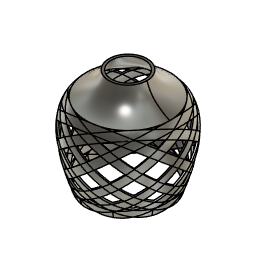
Design a 3D Printed Lampshade_ (Autodesk Fusion 360 design; units mm, degrees)
Autodesk Fusion 360 part; units mm, degrees
sketch "Sketch1" plane through (0, 0, 0) normal (0, 1, 0) x (1, 0, 0)
  line L0 (0, 0) -> (-45, 0)
  line L1 (0, -135) -> (-23.4, -135)
  spline S0 degree 5 poles (-45, 0) (-46.977, -5.2113) (-50.6671, -15.359) (-55.4104, -29.7559) (-60.125, -47.2752) (-63.1831, -66.2213) (-63.2423, -82.0437) (-60.2343, -94.6701) (-54.3436, -104.2914) (-46.1941, -111.555) (-37.1505, -117.879) (-30.513, -123.5506) (-26.5029, -128.8056) (-24.3479, -132.8457) (-23.4, -135) knots 0 0 0 0 0 0 0.1 0.2 0.3 0.4 0.5 0.6 0.7 0.8 0.9 1 1 1 1 1 1
  line L2 (-30, -120) -> (-16.8, -150)
  spline S1 degree 5 poles (-45, 0) (-46.977, -5.2113) (-50.6671, -15.359) (-55.4104, -29.7559) (-60.125, -47.2752) (-63.1831, -66.2213) (-63.2423, -82.0437) (-60.2343, -94.6701) (-54.3436, -104.2914) (-46.1941, -111.555) (-37.1505, -117.879) (-30.513, -123.5506) (-26.5029, -128.8056) (-24.3479, -132.8457) (-23.4, -135) knots 0 0 0 0 0 0 0.1 0.2 0.3 0.4 0.5 0.6 0.7 0.8 0.9 1 1 1 1 1 1
  line L3 (-30, -120) -> (-16.8, -150)
  spline S2 degree 5 poles (-43, 0) (-44.977, -5.2113) (-48.6671, -15.359) (-53.4104, -29.7559) (-58.125, -47.2752) (-61.1831, -66.2213) (-61.2423, -82.0437) (-58.2343, -94.6701) (-52.3436, -104.2914) (-44.1941, -111.555) (-35.1505, -117.879) (-28.513, -123.5506) (-24.5029, -128.8056) (-22.3479, -132.8457) (-21.4, -135) knots 0 0 0 0 0 0 0.1 0.2 0.3 0.4 0.5 0.6 0.7 0.8 0.9 1 1 1 1 1 1
  line L4 (-28, -120) -> (-14.8, -150)
  spline S3 degree 5 poles (-43, 0) (-44.977, -5.2113) (-48.6671, -15.359) (-53.4104, -29.7559) (-58.125, -47.2752) (-61.1831, -66.2213) (-61.2423, -82.0437) (-58.2343, -94.6701) (-52.3436, -104.2914) (-44.1941, -111.555) (-35.1505, -117.879) (-28.513, -123.5506) (-24.5029, -128.8056) (-22.3479, -132.8457) (-21.4, -135) knots 0 0 0 0 0 0 0.1 0.2 0.3 0.4 0.5 0.6 0.7 0.8 0.9 1 1 1 1 1 1
  line L5 (-28, -120) -> (-14.8, -150)
  point P0 (-53.1789, -104.4357)
  point P1 (-53.1789, -104.4357)
  point P2 (-51.1789, -104.4357)
  point P3 (-51.1789, -104.4357)
  constraint coincident L0.start origin
  constraint midpoint L1.end L2
  constraint midpoint L1.end L3
  constraint midpoint S2.end L4
  constraint midpoint S2.end L5
revolve "Revolve1" add sketch "Sketch1" angle 360 about axis through (0, 0, 1.75) along (0, 0, 1) makes body 1
sketch "Sketch2" plane through (0, 0, 0) normal (0, 1, 0) x (1, 0, 0)
  line L0 (-50, -10) -> (70, -110)
  line L1 (70, -110) -> (64.0899, -117.0921)
  line L2 (64.0899, -117.0921) -> (-57.1689, -16.0431)
  line L3 (-57.1689, -16.0431) -> (-50, -10)
  constraint perpendicular L0 L1
  constraint perpendicular L1 L2
extrude "Extrude1" cut sketch "Sketch2" along normal mid plane 240 keep common part bodies 1
pattern_circular "C-Pattern1" count 9 over 360 about axis through (0, 0, 1.75) along (0, 0, 1) of bodies 1 makes body 2 at (42.8106, -42.3489, 63.2494) makes body 3 at (19.4175, -48.7224, 21.1617) makes body 4 at (49.1717, 34.76, 63.2448) makes body 5 at (39.3462, 42.1063, 39.0062) makes body 6 at (3.0756, 57.5466, 39.0062) makes body 7 at (-54.6889, 25.2039, 63.2448) makes body 8 at (-34.9106, 39.1429, 21.1617) makes body 9 at (-46.8826, 21.4455, 18.4185)
sketch "Sketch3" plane through (0, 0, 0) normal (0, 1, 0) x (1, 0, 0)
  line L0 (0, -135) -> (23.4, -135)
  line L1 (51.4013, -106.3579) -> (33.4013, -106.3579)
  spline S0 degree 5 poles (23.4, -135) (24.0607, -132.9354) (25.5161, -129.0744) (28.1011, -124.0867) (32.2406, -118.8224) (38.1836, -113.7797) (43.3152, -110.5) (47.3065, -108.3253) (50.0265, -106.994) (51.4013, -106.3579) knots 0 0 0 0 0 0 0.2 0.4 0.6 0.8 1 1 1 1 1 1
  line L2 (21.8, -140) -> (25, -130)
  spline S1 degree 5 poles (20.4, -135) (21.0607, -132.9354) (22.5161, -129.0744) (25.1011, -124.0867) (29.2406, -118.8224) (35.1836, -113.7797) (40.3152, -110.5) (44.3065, -108.3253) (47.0265, -106.994) (48.4013, -106.3579) knots 0 0 0 0 0 0 0.2 0.4 0.6 0.8 1 1 1 1 1 1
  line L3 (18.8, -140) -> (22, -130)
  constraint horizontal L0
  constraint horizontal L1
  constraint midpoint L0.end L2
  constraint midpoint S1.start L3
revolve "Revolve2" add sketch "Sketch3" angle 360 about axis through (0, 0, 1.75) along (0, 0, 1) separate body makes body 10
